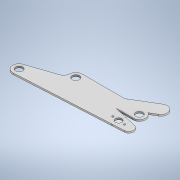
# Autodesk Inventor part: intake-1
Saved by Autodesk Inventor 2022 (Build 260153000, 153)
## iProperties
Created: 2023-01-10
Part Number: intake-1
Material: Generic
Document SubType Name: Modeling
Designer: s135320
Density: 1 g/cm^3
Appearance: Default
Author: s135320
Autodesk Inventor part; units mm, degrees
ref_plane "YZ Plane" through (0, 0, 0) normal (1, 0, 0) x (0, 1, 0)
ref_plane "XZ Plane" through (0, 0, 0) normal (0, 1, 0) x (-1, 0, 0)
ref_plane "XY Plane" through (0, 0, 0) normal (0, 0, 1) x (1, 0, 0)
sketch "Sketch1" plane through (0, 0, 0) normal (0, 1, 0) x (-1, 0, 0)
  line L0 (0, 0) -> (254, 0)
  line L1 (0, -25.4) -> (254, -25.4)
  line L2 (0, 25.4) -> (254, 25.4)
  circle A0 centre (254, 0) radius 25.4
  circle A1 centre (0, 0) radius 25.4
  circle A2 centre (254, 0) radius 14.2875
  circle A3 centre (0, 0) radius 14.2875
  line L3 (76.2, 0) -> (-25.4, -60.8431)
  line L4 (121.5695, -2.4367) -> (-12.3502, -82.6345)
  line L5 (40.7781, 8.3938) -> (-38.4498, -39.0517)
  circle A4 centre (-25.4, -60.8431) radius 25.4
  line L6 (152.4, 0) -> (397.6169, 83.1419)
  line L7 (133.576, 20.4379) -> (389.4609, 107.1969)
  line L8 (172.2557, -20.0881) -> (405.7728, 59.087)
  circle A5 centre (397.6169, 83.1419) radius 25.4
  circle A6 centre (397.6169, 83.1419) radius 14.2875
  circle A7 centre (20.0113, 62.5997) radius 25.4
  line L9 (285.1293, 0) -> (20.0113, 62.5997)
  line L10 (26.7644, 87.1036) -> (18.8052, 88.983)
  line L11 (15.2179, 37.6331) -> (-14.507, 44.6517)
  line L12 (16.2785, 37.4755) -> (15.2179, 37.6331)
  line L13 (27.6621, 86.8201) -> (26.7644, 87.1036)
  line L14 (20.0113, 62.5997) -> (397.6169, 83.1419)
  line L15 (405.4604, 109.0062) -> (-157.3802, 78.387)
  line L16 (-157.3802, 78.387) -> (55.7769, 28.0563)
  line L17 (405.4604, 109.0062) -> (-157.3802, 78.387)
  line L18 (-157.3802, 78.387) -> (92.0162, 19.4994)
  line L19 (417.0671, 58.7625) -> (197.4027, 46.8125)
  line L20 (197.4027, 46.8125) -> (84.4166, 73.4908)
  circle A8 centre (20.0113, 62.5997) radius 12.7
  line L21 (197.4027, 46.8125) -> (-157.3802, 78.387)
  circle A9 centre (-5.2887, 64.8513) radius 3.4925
  circle A10 centre (45.3113, 60.3481) radius 3.4925
  point P0 (107.1023, -119.4279)
  point P1 (83.2238, -25.4)
  point P2 (2.9551, -25.4)
  point P3 (148.2111, 25.4)
  point P4 (236.1593, 25.4)
  point P5 (274.7421, 14.6604)
  point P6 (-11.2587, -22.7684)
  point P7 (16.3526, 37.9742)
  point P8 (0.338, 25.4)
  point P9 (70.7471, 25.4)
  point P10 (25.8482, 87.3199)
  point P11 (27.8621, 87.4532)
  point P12 (0.3401, 25.3977)
  point P13 (17.5299, 80.8522)
  point P14 (214.0328, 47.7172)
  point P15 (396.2371, 108.5044)
  point P16 (18.6315, 87.9622)
  point P17 (-4.7407, 68.3006)
  point P18 (14.1743, 37.8795)
  point P19 (-5.3584, 61.3595)
  point P20 (22.2862, 88.161)
  point P21 (87.1938, 73.6518)
  point P22 (44.7633, 56.8989)
  point P23 (44.7315, 56.7628)
  point P24 (160.2581, 29.4846)
  point P25 (45.381, 63.8399)
  point P26 (402.4744, 57.9686)
  point P27 (398.9966, 57.7794)
  point P28 (308.2536, 52.8429)
  point P29 (227.3142, 25.4)
  point P30 (177.5569, 25.4)
  point P31 (55.7769, 28.0563)
  point P32 (67.0265, 25.4)
  dimension "d0" = 25.4
  dimension "d1" = 25.4
  dimension "d2" = 28.575
  dimension "d3" = 28.575
  dimension "d6" = 254
  dimension "d7" = 76.2
  dimension "d8" = 25.4
  dimension "d9" = 25.4
  dimension "d11" = 50.8
  dimension "d13" = 25.4
  dimension "d14" = 25.4
  dimension "d15" = 50.8
  dimension "d16" = 101.6
  dimension "d18" = 28.575
  dimension "d23" = 50.8
  dimension "d24" = 25.4
  dimension "d25" = 25.4
  dimension "d26" = 25.4
  dimension "d27" = 25.4
  dimension "d28" = 25.4
  dimension "d29" = 25.4
  dimension "d30" = 6.985
  dimension "d31" = 6.985
  constraints: 44 end point, 12 point on circle, 11 centre point, 8 coincident, 6 parallel, 5 point on line, 4 tangent, 1 horizontal, 3 other
  measures "d0" distance between parallel lines of L0 L2
  measures "d1" distance between parallel lines of L1 L0
  measures "d2" diameter of A3
  measures "d3" diameter of A2
  measures "d6" distance of L0.start L0.end
  measures "d7" distance of L0.start L3.start
  measures "d8" distance between parallel lines of L3 L4
  measures "d9" distance between parallel lines of L3 L5
  measures "d11" diameter of A4
  measures "d13" distance between parallel lines of L6 L7
  measures "d14" distance between parallel lines of L6 L8
  measures "d15" diameter of A5
  measures "d16" distance of L0.end L6.start
  measures "d18" diameter of A6
  measures "d23" diameter of A7
  measures "d24" distance between parallel lines of L9 L10
  measures "d25" distance between parallel lines of L9 L11
  measures "d26" distance between parallel lines of L14 L15
  measures "d27" distance between parallel lines of L14 L17
  measures "d28" distance between parallel lines of L14 L19
  measures "d29" diameter of A8
  measures "d30" diameter of A9
  measures "d31" diameter of A10
extrude "Extrusion1" add sketch "Sketch1" along normal blind 6.35 contours A3 L5 A1 L0 | L0 A1 L5 A3 | A1 L2 L9 L6 L0 | L0 L5 A1 | A3 L5 A1 | L0 L3 L1 A1 L5 | A1 L1 L3 A4 L5 | L0 A0 L1 L3 | L18 L16 L12 A7 L9 L7 L2 | A4 | L6 L9 A0 L0 | L1 L4 A4 L3 | L7 L9 L2 | A0 L9 A2 L8 L0 | L0 L8 A0 | L9 L2 L6 | L6 L2 A0 L9 | L9 L7 L19 L6 L2 | L9 A7 A10 L21 L19 L7 | L8 A2 L0 | L0 A2 L9 A0 L8 | A0 L8 A2 L9 | L6 L19 L8 A0 L2 | L19 L20 L14 L7 | L7 L14 A5 L6 L19 | L9 A8 L21 A10 A7 | A7 A9 L21 A8 L9 | L11 L16 L21 A9 A7 | L6 A5 L19 | L14 A7 L13 L10 L15 A5 L7 | L7 A5 L14 | L21 A10 A7 L14 L20 | A10 L21 A7 | A8 L21 L9 | L9 L21 A8 | A7 L21 A9 | A0 L9 A2 L8 | A5 L14 A6 L6 | L6 A6 L14 A5 | L21 A10 A7 | L21 A8 L14 A7 A10 | L21 A8 L14 | L14 A8 L21 | L21 A9 A7 L14 A8 | A7 A9 L21 | L21 L15 A7 A9 | A7 L10 L13 picked at (44.1131, 59.8161) picked at (-4.2032, 64.1161) picked at (43.0407, 60.7991) picked at (-4.1134, 65.5089)
fillet "Fillet1" radius 25.4 2 edges at (-83.2238, 3.175, -25.4) (-274.7421, 3.175, 14.6604)
sketch "Sketch2" plane through (0, 0, 0) normal (0, -1, 0) x (1, 0, 0)
  circle A0 centre (-254, 0) radius 14.2875 projected
  arc A1 (-197.2039, -50.8) -> (-177.8, 0) centre (-254, 0) ccw
  line L0 (-254, 0) -> (-197.2039, -50.8)
  point P0 (0, 0)
  dimension "d19" = 76.2
  dimension "d20" = 50.8
  constraints: 2 end point, 2 point on circle, 1 centre point, 1 coincident
  measures "d19" radius of A1
  measures "d20" vertical distance of L0.start L0.end
extrude "Extrusion2" cut sketch "Sketch1" along normal through all contours A10 L21 A7 | A7 L21 A10 | A8 L21 L9 | L9 L21 A8 | A7 L21 A9 | L21 A7 A10 | L21 A10 A7 | L21 A8 L14 | L14 A8 L21 | A7 A9 L21 picked at (-4.2032, 64.1161) picked at (-4.1134, 65.5089)
fillet "Fillet2" radius 19.05 1 edges at (157.3802, 3.175, 78.387)
equation "\"d0\" = d1"
body "Solid1"
